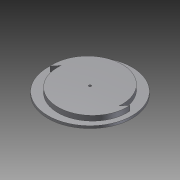
# Autodesk Inventor part: Rueda superior
Saved by Autodesk Inventor 2011 (Build 150239000, 239)
## iProperties
Created: 2014-08-05
Part Number: Rueda superior
Document SubType Name: Modeling
Designer: Admin
Density: 1 g/cm^3
Author: Admin
Autodesk Inventor part; units mm, degrees
ref_plane "YZ Plane" through (0, 0, 0) normal (1, 0, 0) x (0, 1, 0)
ref_plane "XZ Plane" through (0, 0, 0) normal (0, 1, 0) x (-1, 0, 0)
ref_plane "XY Plane" through (0, 0, 0) normal (0, 0, 1) x (1, 0, 0)
sketch "Boceto1" plane through (0, 0, 0) normal (0, 0, 1) x (1, 0, 0)
  circle A0 centre (0, 0) radius 17
  circle A1 centre (0, 0) radius 0.5
  dimension "d0" = 34
  dimension "d1" = 1
  constraints: 2 centre point, 1 coincident, 1 concentric
  measures "d0" diameter of A0
  measures "d1" diameter of A1
extrude "Extrusión1" add sketch "Boceto1" along normal blind 1
sketch "Boceto2" plane through (0, 0, 1) normal (0, 0, 1) x (1, 0, 0)
  circle A0 centre (0, 0) radius 0.5 projected
  circle A1 centre (0, 0) radius 17 projected
  line L0 (0, 0) -> (20, 0) construction
  line L1 (0, 0) -> (20, 0) construction
  arc A2 (13, 0) -> (-15, 0) centre (-1, -0.0014) ccw
  arc A3 (12.9468, -1.2202) -> (13, 0) centre (-1, -0.0014) ccw
  line L2 (13, 0) -> (-1, -0.0014) construction
  line L3 (12.9468, -1.2202) -> (-1, -0.0014) construction
  arc A4 (-15, 0) -> (-14.9468, -1.2202) centre (-1, -0.0014) ccw
  line L4 (-15, 0) -> (-1, -0.0014) construction
  line L5 (-14.9468, -1.2202) -> (-1, -0.0014) construction
  arc A5 (-13, 0) -> (15, 0) centre (1, 0.0014) ccw
  arc A6 (-12.9468, 1.2202) -> (-13, 0) centre (1, 0.0014) ccw
  line L6 (-13, 0) -> (1, 0.0014) construction
  line L7 (-12.9468, 1.2202) -> (1, 0.0014) construction
  arc A7 (15, 0) -> (14.9468, 1.2202) centre (1, 0.0014) ccw
  line L8 (15, 0) -> (1, 0.0014) construction
  line L9 (14.9468, 1.2202) -> (1, 0.0014) construction
  line L10 (-12.9468, 1.2202) -> (-14.9468, -1.2202)
  line L11 (12.9468, -1.2202) -> (14.9468, 1.2202)
  dimension "d15" = 28
  dimension "d16" = 14
  dimension "d18" = 14
  dimension "d19" = 5
  dimension "d20" = 14
  dimension "d21" = 5
  dimension "d24" = 360
  dimension "d26" = 15
  constraints: 24 end point, 12 point on circle, 6 centre point, 2 concentric, 2 horizontal, 2 point on line, 1 parallel, 29 other
  measures "d15" distance of L2.start L4.start
  measures "d16" radius of A2
  measures "d18" radius of A3
  measures "d19" angle of L3 L2
  measures "d20" radius of A4
  measures "d21" angle of L4 L5
  measures "d26" distance of L4.start A0.centre
extrude "Extrusión2" add sketch "Boceto2" along normal blind 2 contours A3 L11 A7 A5 A6 L10 A4 A2
